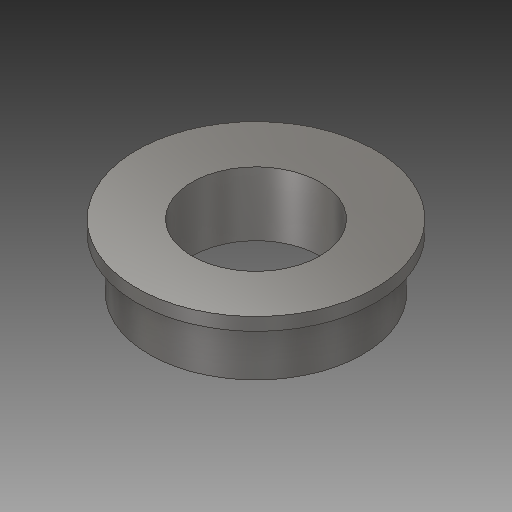
# Autodesk Inventor part: ベアリングフランジ付き0610.3t
Saved by Autodesk Inventor 2020 (Build 240168000, 168)
## iProperties
Part Number: ベアリングフランジ付き0610.3t
Material: ステンレス鋼
Document SubType Name: Modeling
Designer: 雪村
Density: 8 g/cm^3
Appearance: 半つや出し
Mass: 1.30228 g
Surface Area: 2.9355 cm^2
Volume: 0.162785 cm^3
Author: 雪村
Autodesk Inventor part; units mm, degrees
ref_plane "YZ Plane" through (0, 0, 0) normal (1, 0, 0) x (0, 1, 0)
ref_plane "XZ Plane" through (0, 0, 0) normal (0, 1, 0) x (-1, 0, 0)
ref_plane "XY Plane" through (0, 0, 0) normal (0, 0, 1) x (1, 0, 0)
sketch "スケッチ1" plane through (0, 0, 0) normal (0, 1, 0) x (-1, 0, 0)
  circle A0 centre (0, 0) radius 3
  circle A1 centre (0, 0) radius 5
  dimension "d0" = 6
  dimension "d1" = 10
  constraints: 2 centre point, 2 coincident
  measures "d0" diameter of A0
  measures "d1" diameter of A1
extrude "押し出し1" add sketch "スケッチ1" along normal blind 3
sketch "スケッチ2" plane through (0, 3, 0) normal (0, 1, 0) x (1, 0, 0)
  circle A0 centre (0, 0) radius 3 projected
  circle A1 centre (0, 0) radius 5 projected
  circle A2 centre (0, 0) radius 5.6
  dimension "d4" = 11.2
  constraints: 1 centre point, 1 coincident
  measures "d4" diameter of A2
extrude "押し出し2" add sketch "スケッチ2" against normal blind 0.6 contours A1 | A2
